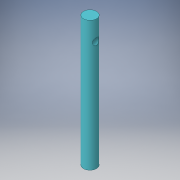
# Autodesk Inventor part: Lower Half of Clutch
Saved by Autodesk Inventor 2016 (Build 200138000, 138)
## iProperties
Created: 2015-06-15
Part Number: Lower Half of Clutch
Material: Aluminum 6061
Document SubType Name: Modeling
Designer: steele
Density: 2.7 g/cm^3
Appearance: Cadet Blue
Author: steele
Autodesk Inventor part; units mm, degrees
ref_plane "XZ Plane" through (0, 0, 0) normal (0, 1, 0) x (-1, 0, 0)
ref_plane "XY Plane" through (0, 0, 0) normal (0, 0, 1) x (1, 0, 0)
sketch "Sketch1" plane through (0, 0, 0) normal (0, 1, 0) x (-1, 0, 0)
  circle A0 centre (0, 0) radius 6.35
  dimension "d0" = 12.7
  constraints: 1 centre point, 1 coincident
  measures "d0" diameter of A0
extrude "Extrusion1" add sketch "Sketch1" against normal blind 127
ref_plane "Work Plane1" through (6.35, 0, 0) normal (1, 0, 0) x (0, 1, 0)
sketch "Sketch3" plane through (6.35, 0, 0) normal (1, 0, 0) x (0, 1, 0)
  line L0 (0, 6.35) -> (-127, 6.35) construction
  line L1 (-19.05, 6.35) -> (-19.05, -6.35) construction
  line L2 (0, -6.35) -> (-127, -6.35) construction
  line L3 (0, 6.35) -> (0, -6.35) construction
  circle A0 centre (-19.05, 0) radius 3.302
  point P0 (0, 0)
  dimension "d4" = 19.05
  dimension "d5" = 6.604
  constraints: 2 end point, 2 point on line, 1 centre point, 1 midpoint, 1 vertical
  measures "d4" distance between parallel lines of L1 L3
  measures "d5" diameter of A0
extrude "Extrusion2" cut sketch "Sketch3" against normal through all
body "Solid1"
